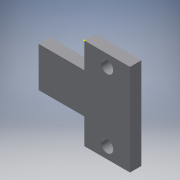
# Autodesk Inventor part: IC slider
Saved by Autodesk Inventor 2018 (Build 220112000, 112)
## iProperties
Created: 2018-02-03
Part Number: IC slider
Material: Generic
Document SubType Name: Modeling
Designer: Luke
Density: 1 g/cm^3
Appearance: Default
Author: Luke
Autodesk Inventor part; units mm, degrees
ref_plane "YZ Plane" through (0, 0, 0) normal (1, 0, 0) x (0, 1, 0)
ref_plane "XZ Plane" through (0, 0, 0) normal (0, 1, 0) x (-1, 0, 0)
ref_plane "XY Plane" through (0, 0, 0) normal (0, 0, 1) x (1, 0, 0)
sketch "Sketch1" plane through (0, 0, 0) normal (0, 0, 1) x (1, 0, 0)
  line L0 (0, 0) -> (50.8, 0)
  line L1 (50.8, 0) -> (50.8, -152.4)
  line L2 (50.8, -152.4) -> (0, -152.4)
  line L3 (0, -152.4) -> (0, 0)
  circle A0 centre (25.4, -114.3) radius 6.731
  circle A1 centre (25.4, -38.1) radius 6.731
  dimension "d0" = 50.8
  dimension "d1" = 152.4
  dimension "d2" = 13.462
  dimension "d3" = 13.462
  dimension "d4" = 25.4
  dimension "d5" = 25.4
  dimension "d6" = 38.1
  dimension "d7" = 38.1
  constraints: 8 end point, 2 centre point, 2 parallel, 1 horizontal, 1 perpendicular
  measures "d0" distance of L1.end L2.end
  measures "d1" distance of L0.end L1.end
  measures "d2" diameter of A1
  measures "d3" diameter of A0
  measures "d4" distance from line of L1 A0.centre
  measures "d5" distance from line of L1 A1.centre
  measures "d6" distance from line of L0 A1.centre
  measures "d7" distance from line of L2 A0.centre
extrude "Extrusion1" add sketch "Sketch1" along normal blind 12.7
sketch "Sketch3" plane through (0, 0, 12.7) normal (0, 0, 1) x (1, 0, 0)
  point P0 (0, 0)
sketch "Sketch4" plane through (0, 0, 12.7) normal (0, 0, 1) x (1, 0, 0)
  line L0 (0, 0) -> (0, -152.4) projected
  line L1 (0, -47.625) -> (-50.8, -47.625)
  line L2 (-50.8, -47.625) -> (-50.8, -92.075)
  line L3 (-50.8, -92.075) -> (0, -92.075)
  line L4 (0, -92.075) -> (0, -47.625)
  line L5 (0, -152.4) -> (50.8, -152.4) projected
  dimension "d23" = 50.8
  dimension "d24" = 44.45
  dimension "d27" = 104.775
  constraints: 8 end point, 2 parallel, 1 horizontal, 1 perpendicular, 1 point on line
  measures "d23" distance of L1.start L1.end
  measures "d24" distance between parallel lines of L1 L3
  measures "d27" distance between parallel lines of L5 L1
extrude "Extrusion3" add sketch "Sketch4" against normal blind 12.7
body "Solid1"
